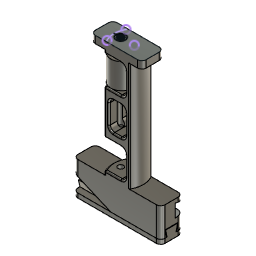
dual_mount_rolling_spool (Autodesk Fusion 360 design; units mm, degrees)
Autodesk Fusion 360 part; units mm, degrees
note: some values were not read from the file. Chosen so that the rebuilt part matches the saved one: which face or edge a step refers to.
sketch "Sketch1" plane through (0, 0, 0) normal (0, 0, 1) x (1, 0, 0)
  line L0 (0, 0) -> (60, 0)
  line L1 (60, 0) -> (60, 15)
  line L2 (60, 15) -> (0, 15)
  line L3 (0, 15) -> (0, 0)
  dimension "d1" = 60
  dimension "d2" = 15
  constraint horizontal L0
  constraint vertical L1
  constraint horizontal L2
  constraint vertical L3
  constraint coincident L0.start L3.end
  measures "d1" distance of L0.start L0.end
  measures "d2" distance of L0.start L2.end
extrude "Extrude1" add sketch "Sketch1" along normal blind 10 makes body 1
sketch "Sketch2" plane through (0, 0, 10) normal (0, 0, 1) x (-1, 0, 0)
  line L0 (0, -15) -> (0, 0)
  line L1 (0, 0) -> (-60, 0)
  line L2 (-60, 0) -> (-60, -15)
  line L3 (-60, -15) -> (0, -15)
  line L4 (-40.5, 0) -> (-19.5, 0)
  line L5 (-19.5, 0) -> (-19.5, -15)
  line L6 (-19.5, -15) -> (-40.5, -15)
  line L7 (-40.5, -15) -> (-40.5, 0) construction
  line L8 (-40.5, 0) -> (-19.5, -15) construction
  line L9 (-19.5, 0) -> (-40.5, -15) construction
  line L10 (-38.4665, -15) -> (-38.4665, 0) construction
  arc A0 (-38.4665, 0) -> (-38.4665, -15) centre (-25.6527, -7.5) ccw
  line L11 (-30, -7.5) -> (-30, -10.6) construction
  arc A1 (-21.5335, -15) -> (-21.5335, 0) centre (-34.3473, -7.5) ccw
  point P0 (-30, -7.5)
  dimension "d5" = 21
  constraint horizontal L4
  constraint perpendicular L4 L5
  constraint parallel L4 L6
  constraint parallel L5 L7
  constraint coincident L8 P0
  constraint coincident L9 P0
  constraint vertical L10
  constraint coincident L6 L10.start
  constraint coincident L3 L10.start
  constraint coincident L4 L10.end
  constraint coincident L1 L10.end
  constraint tangent L7 A0
  constraint coincident P0 L11.start
  constraint vertical L11
  constraint symmetric L10.start L11 A1.start
  constraint symmetric L10.end L11 A1.end
  constraint symmetric A0 L11 A1
  measures "d5" distance of L5.end L6.end
extrude "Extrude2" add sketch "Sketch2" along normal blind 75 contours L1 L3 L4 L6 A0 A1 bodies 1
fillet "Fillet1" radius 1 4 edges at (38.4665, 15, 47.5) (21.5335, 15, 47.5) (38.4665, 0, 47.5) (21.5335, 0, 47.5) on bodies 1
fillet "Fillet2" radius 3 4 edges at (60, 15, 5) (60, 0, 5) (0, 15, 5) (0, 0, 5) on bodies 1
sketch "Sketch3" plane through (0, 15, 0) normal (0, 1, 0) x (-1, 0, 0)
  line L0 (-3, 0) -> (-3, 10)
  line L1 (-3, 10) -> (-22.1204, 10)
  line L2 (-22.1204, 10) -> (-22.1204, 85)
  line L3 (-22.1204, 85) -> (-37.8796, 85)
  line L4 (-37.8796, 85) -> (-37.8796, 10)
  line L5 (-37.8796, 10) -> (-57, 10)
  line L6 (-57, 10) -> (-57, 0)
  line L7 (-57, 0) -> (-3, 0)
  line L8 (-22.1204, 10) -> (-22.1204, 35) construction
  line L9 (-22.1204, 35) -> (-22.1204, 60) construction
  line L10 (-27.4, 37.8) -> (-32.6, 37.8)
  line L11 (-35.6, 40.8) -> (-35.6, 54.2)
  line L12 (-32.6, 57.2) -> (-27.4, 57.2)
  line L13 (-24.4, 54.2) -> (-24.4, 40.8)
  line L14 (-24.4, 37.8) -> (-35.6, 57.2) construction
  line L15 (-35.6, 37.8) -> (-24.4, 57.2) construction
  arc A0 (-32.6, 57.2) -> (-35.6, 54.2) centre (-32.6, 54.2) ccw
  arc A1 (-24.4, 54.2) -> (-27.4, 57.2) centre (-27.4, 54.2) ccw
  arc A2 (-35.6, 40.8) -> (-32.6, 37.8) centre (-32.6, 40.8) ccw
  arc A3 (-27.4, 37.8) -> (-24.4, 40.8) centre (-27.4, 40.8) ccw
  line L16 (-22.1204, 35) -> (-24.6, 35) construction
  line L17 (-22.1204, 60) -> (-24.4, 60) construction
  line L18 (-24.4, 65.8) -> (-24.4, 79.2)
  arc A4 (-27.4, 62.8) -> (-24.4, 65.8) centre (-27.4, 65.8) ccw
  line L19 (-32.6, 62.8) -> (-27.4, 62.8)
  arc A5 (-35.6, 65.8) -> (-32.6, 62.8) centre (-32.6, 65.8) ccw
  line L20 (-35.6, 79.2) -> (-35.6, 65.8)
  arc A6 (-32.6, 82.2) -> (-35.6, 79.2) centre (-32.6, 79.2) ccw
  line L21 (-27.4, 82.2) -> (-32.6, 82.2)
  arc A7 (-24.4, 79.2) -> (-27.4, 82.2) centre (-27.4, 79.2) ccw
  line L22 (-27.4, 32.2) -> (-32.6, 32.2)
  arc A8 (-24.4, 29.2) -> (-27.4, 32.2) centre (-27.4, 29.2) ccw
  line L23 (-24.4, 15.8) -> (-24.4, 29.2)
  arc A9 (-32.6, 32.2) -> (-35.6, 29.2) centre (-32.6, 29.2) ccw
  line L24 (-35.6, 29.2) -> (-35.6, 15.8)
  line L25 (-32.6, 12.8) -> (-27.4, 12.8)
  arc A10 (-27.4, 12.8) -> (-24.4, 15.8) centre (-27.4, 15.8) ccw
  arc A11 (-35.6, 15.8) -> (-32.6, 12.8) centre (-32.6, 15.8) ccw
  line L26 (-19.5, 85) -> (-21.2374, 85)
  line L27 (-19.5, 85) -> (-19.5, 10)
  line L28 (-30, 12.8) -> (-19.5, 12.8)
  line L29 (-30, 32.2) -> (-19.5, 32.2)
  line L30 (-19.5, 12.8) -> (-19.5, 32.2)
  line L31 (-30, 62.8) -> (-19.5, 62.8)
  line L32 (-30, 82.2) -> (-19.5, 82.2)
  point P0 (-30, 47.5)
  dimension "d12" = 25
  dimension "d13" = 25
  dimension "d14" = 3
  dimension "d15" = 3
  dimension "d16" = 3
  dimension "d17" = 3
  constraint coincident L1.end L2.start
  constraint perpendicular L3 L8
  constraint parallel L2 L9
  constraint horizontal L10
  constraint perpendicular L10 L11
  constraint parallel L10 L12
  constraint parallel L11 L13
  constraint coincident L14 P0
  constraint coincident L15 P0
  constraint coincident L14.end L12
  constraint coincident L14.end L11
  constraint tangent L12 A0
  constraint tangent L11 A0
  constraint coincident L15.end L12
  constraint coincident L15.end L13
  constraint tangent L12 A1
  constraint tangent L13 A1
  constraint coincident L15.start L11
  constraint coincident L15.start L10
  constraint tangent L11 A2
  constraint tangent L10 A2
  constraint coincident L14.start L13
  constraint coincident L14.start L10
  constraint tangent L13 A3
  constraint tangent L10 A3
  constraint perpendicular L2 L16
  constraint perpendicular L2 L17
  constraint symmetric L12.start L17 L19.start
  constraint symmetric L11.end L17 A5.start
  constraint symmetric A0 L17 A5
  constraint symmetric L12.end L17 A4.start
  constraint symmetric L13.start L17 L18.start
  constraint symmetric A1 L17 A4
  constraint symmetric L11.start L17 L20.start
  constraint symmetric L10.end L17 A6.start
  constraint symmetric A2 L17 A6
  constraint symmetric L13.end L17 L18.end
  constraint symmetric L10.start L17 L21.start
  constraint symmetric A3 L17 A7
  constraint symmetric L12.start L16 L25.start
  constraint symmetric L11.end L16 L24.end
  constraint symmetric A0 L16 A11
  constraint symmetric L12.end L16 L25.end
  constraint symmetric L13.start L16 L23.start
  constraint symmetric A1 L16 A10
  constraint symmetric L11.start L16 A9.end
  constraint symmetric L10.end L16 L22.end
  constraint symmetric A2 L16 A9
  constraint symmetric L13.end L16 A8.start
  constraint symmetric L10.start L16 L22.start
  constraint symmetric A3 L16 A8
  constraint coincident L26.start L27.start
  constraint coincident L1 L27.end
  constraint perpendicular L1 L27
  constraint midpoint L25 L28.start
  constraint coincident L27 L28.end
  constraint perpendicular L27 L28
  constraint midpoint L22 L29.start
  constraint coincident L27 L29.end
  constraint perpendicular L27 L29
  constraint midpoint L19 L31.start
  constraint coincident L27 L31.end
  constraint perpendicular L27 L31
  constraint midpoint L21 L32.start
  constraint coincident L27 L32.end
  constraint perpendicular L27 L32
  measures "d12" distance of L1.end L8.end
  measures "d13" distance of L8.end L9.end
  measures "d14" radius of A0
  measures "d15" radius of A1
  measures "d16" radius of A2
  measures "d17" radius of A3
extrude "Extrude6" cut sketch "Sketch3" against normal blind 15 contours L2 L27 L28 L29 L30 | L2 A8 L23 A10 L28 L29 | L2 L27 L31 L32 | L2 L18 A4 A7 L31 L32 bodies 1
extrude "Extrude3" cut sketch "Sketch3" against normal blind 15 contours L22 A8 L23 A9 L24 L25 A10 A11 L28 L29 | L18 A4 L19 A5 L20 A6 L21 A7 L31 L32 | L10 L11 L12 L13 A0 A1 A2 A3 bodies 1
fillet "Fillet3" radius 1 48 edges at (27.3602, 15, 82.2) (34.7213, 15, 81.3213) (35.6, 15, 72.5) (34.7213, 15, 63.6787) (27.3602, 15, 62.8) (27.3602, 15, 32.2) (34.7213, 15, 31.3213) (35.6, 15, 22.5) (34.7213, 15, 13.6787) (27.3602, 15, 12.8) (30, 15, 37.8) (25.2787, 15, 38.6787) (24.4, 15, 47.5) (25.2787, 15, 56.3213) (30, 15, 57.2) (34.7213, 15, 56.3213) (35.6, 15, 47.5) (34.7213, 15, 38.6787) (21.6053, 14.8571, 12.8) (21.6053, 0.1429, 12.8) (19.5, 7.5, 12.8) (27.3602, 0, 12.8) (34.7213, 0, 13.6787) (35.6, 0, 22.5) (34.7213, 0, 31.3213) (21.6053, 14.8571, 32.2) (19.5, 7.5, 32.2) (21.6053, 0.1429, 32.2) (27.3602, 0, 32.2) (21.6053, 14.8571, 62.8) (27.3602, 0, 62.8) (21.6053, 0.1429, 62.8) (19.5, 7.5, 62.8) (34.7213, 0, 63.6787) (35.6, 0, 72.5) (34.7213, 0, 81.3213) (21.6053, 14.8571, 82.2) (19.5, 7.5, 82.2) (21.6053, 0.1429, 82.2) (27.3602, 0, 82.2) (30, 0, 37.8) (34.7213, 0, 38.6787) (35.6, 0, 47.5) (34.7213, 0, 56.3213) (30, 0, 57.2) (25.2787, 0, 56.3213) (24.4, 0, 47.5) (25.2787, 0, 38.6787) on bodies 1
sketch "Sketch4" plane through (0, 0, 10) normal (0, 0, 1) x (-1, 0, 0)
  arc A0 (-57, 0) -> (-60, -3) centre (-57, -3) ccw
  line L0 (-60, -3) -> (-60, -12)
  arc A1 (-60, -12) -> (-57, -15) centre (-57, -12) ccw
  line L1 (-57, -15) -> (-37.8796, -15)
  arc A2 (-38.7626, -14.4694) -> (-37.8796, -15) centre (-37.8796, -14) ccw
  arc A3 (-38.7626, -0.5306) -> (-38.7626, -14.4694) centre (-25.6527, -7.5) ccw
  arc A4 (-37.8796, 0) -> (-38.7626, -0.5306) centre (-37.8796, -1) ccw
  line L2 (-37.8796, 0) -> (-57, 0)
  line L3 (-60, -7.5) -> (-55, -7.5)
  circle A5 centre (-51.8, -7.5) radius 3.2
  circle A6 centre (-51.8, -7.5) radius 1.9
  dimension "d22" = 5
  dimension "d23" = 6.4
  dimension "d24" = 3.8
  constraint midpoint L0 L3.start
  constraint perpendicular L0 L3
  constraint coincident L3.end A5
  constraint concentric A5 A6
  measures "d22" distance of L3.start L3.end
  measures "d23" diameter of A5
  measures "d24" diameter of A6
extrude "Extrude4" [suppressed]
extrude "Extrude5" [suppressed]
ref_plane "WorkPlane1" through (30, 7.5, 5) normal (1, 0, 0) x (0, 1, 0)
mirror "Mirror1" [suppressed]
sketch "Sketch5" plane through (0, 0, 85) normal (0, 0, 1) x (-1, 0, 0)
  arc A0 (-21.2374, -0.5306) -> (-22.1204, 0) centre (-22.1204, -1) ccw
  line L0 (-22.1204, 0) -> (-37.8796, 0)
  arc A1 (-37.8796, 0) -> (-38.7626, -0.5306) centre (-37.8796, -1) ccw
  arc A2 (-38.7626, -0.5306) -> (-38.7626, -14.4694) centre (-25.6527, -7.5) ccw
  arc A3 (-38.7626, -14.4694) -> (-37.8796, -15) centre (-37.8796, -14) ccw
  line L1 (-37.8796, -15) -> (-22.1204, -15)
  arc A4 (-22.1204, -15) -> (-21.2374, -14.4694) centre (-22.1204, -14) ccw
  arc A5 (-21.2374, -14.4694) -> (-21.2374, -0.5306) centre (-34.3473, -7.5) ccw
  line L2 (-30, -15) -> (-47, -15)
  line L3 (-44, -15) -> (-15, -15)
  line L4 (-12, -12) -> (-12, -3)
  line L5 (-15, 0) -> (-44, 0)
  line L6 (-47, -3) -> (-47, -12)
  arc A6 (-15, -15) -> (-12, -12) centre (-15, -12) ccw
  arc A7 (-12, -3) -> (-15, 0) centre (-15, -3) ccw
  arc A8 (-47, -12) -> (-44, -15) centre (-44, -12) ccw
  arc A9 (-44, 0) -> (-47, -3) centre (-44, -3) ccw
  point P0 (-12, -15)
  dimension "d34" = 17
  dimension "d35" = 35
  dimension "d36" = 3
  dimension "d37" = 3
  dimension "d38" = 3
  dimension "d39" = 3
  constraint midpoint L1 L2.start
  constraint parallel L1 L2
  constraint horizontal L3
  constraint vertical L4
  constraint horizontal L5
  constraint vertical L6
  constraint coincident P0 L3
  constraint coincident P0 L4
  constraint tangent L3 A6
  constraint tangent L4 A6
  constraint tangent L4 A7
  constraint tangent L5 A7
  constraint coincident L2.end L6
  constraint coincident L2.end L3
  constraint tangent L6 A8
  constraint tangent L3 A8
  constraint tangent L6 A9
  constraint tangent L5 A9
  measures "d34" distance of L2.start L2.end
  measures "d35" distance of L2.end P0
  measures "d36" radius of A6
  measures "d37" radius of A7
  measures "d38" radius of A8
  measures "d39" radius of A9
extrude "Extrude7" add sketch "Sketch5" along normal blind 5 bodies 1
sketch "Sketch6" plane through (0, 0, 90) normal (0, 0, 1) x (-1, 0, 0)
  arc A0 (-44, 0) -> (-47, -3) centre (-44, -3) ccw
  line L0 (-47, -3) -> (-47, -12)
  arc A1 (-47, -12) -> (-44, -15) centre (-44, -12) ccw
  line L1 (-44, -15) -> (-15, -15)
  arc A2 (-15, -15) -> (-12, -12) centre (-15, -12) ccw
  line L2 (-12, -12) -> (-12, -3)
  arc A3 (-12, -3) -> (-15, 0) centre (-15, -3) ccw
  line L3 (-15, 0) -> (-44, 0)
  arc A4 (-22.1204, -14) -> (-22.1204, -1) centre (-34.3473, -7.5) ccw
  line L4 (-20.5, -7.5) -> (-25, -7.5)
  circle A5 centre (-25, -7.5) radius 1.9
  circle A6 centre (-25, -7.5) radius 3.2
  dimension "d42" = 4.5
  dimension "d43" = 3.8
  dimension "d44" = 6.4
  constraint midpoint A4 L4.start
  constraint horizontal L4
  constraint coincident L4.end A5.centre
  measures "d42" distance of L4.start L4.end
  measures "d43" diameter of A5
  measures "d44" diameter of A6
extrude "Extrude8" cut sketch "Sketch6" against normal blind 90 contours A5 bodies 1
extrude "Extrude9" cut sketch "Sketch6" against normal blind 1.5 contours A6 bodies 1
sketch "Sketch7" plane through (0, 0, 0) normal (0, 0, -1) x (1, 0, 0)
  circle A0 centre (25, -7.5) radius 1.9
  arc A1 (3, 0) -> (0, -3) centre (3, -3) ccw
  line L0 (0, -3) -> (0, -12)
  arc A2 (0, -12) -> (3, -15) centre (3, -12) ccw
  line L1 (3, -15) -> (57, -15)
  arc A3 (57, -15) -> (60, -12) centre (57, -12) ccw
  line L2 (60, -12) -> (60, -3)
  arc A4 (60, -3) -> (57, 0) centre (57, -3) ccw
  line L3 (57, 0) -> (3, 0)
  circle A5 centre (25, -7.5) radius 3.2
  dimension "d49" = 6.4
  constraint concentric A0 A5
  measures "d49" diameter of A5
extrude "Extrude10" [suppressed]
sketch "Sketch8" plane through (0, 0, 0) normal (1, 0, 0) x (0, 1, 0)
  line L0 (1, 62.8) -> (14, 62.8)
  line L1 (14, 57.2) -> (1, 57.2)
  line L2 (7.5, 57.2) -> (7.5, 62.8) construction
  line L3 (4.65, 61.6) -> (10.35, 61.6)
  line L4 (10.35, 61.6) -> (10.35, 58.4)
  line L5 (10.35, 58.4) -> (4.65, 58.4)
  line L6 (4.65, 58.4) -> (4.65, 61.6)
  line L7 (4.65, 61.6) -> (10.35, 58.4) construction
  line L8 (10.35, 61.6) -> (4.65, 58.4) construction
  point P0 (7.5, 60)
  dimension "d52" = 5.7
  dimension "d53" = 3.2
  constraint midpoint L1 L2.start
  constraint midpoint L0 L2.end
  constraint horizontal L3
  constraint perpendicular L3 L4
  constraint parallel L3 L5
  constraint parallel L4 L6
  constraint coincident L7 P0
  constraint coincident L8 P0
  constraint midpoint L2 P0
  measures "d52" distance of L4.end L5.end
  measures "d53" distance of L3.end L4.end
extrude "Extrude11" cut sketch "Sketch8" along normal blind 28.9 bodies 1
ref_plane "WorkPlane2" through (25.6324, 7.5, 47.5) normal (0, 0, 1) x (-1, 0, 0)
mirror "Mirror2" about plane through (25.6324, 7.5, 47.5) normal (0, 0, 1) of "Extrude11"
ref_plane "WorkPlane3" through (25.6324, 7.5, 63.8) normal (0, 0, 1) x (-1, 0, 0)
sketch "Sketch9" plane through (25.6324, 7.5, 63.8) normal (0, 0, 1) x (1, 0, 0)
  circle A0 centre (0, 0) radius 7.5
  circle A1 centre (0, 0) radius 2
  dimension "d60" = 15
  dimension "d61" = 4
  constraint coincident A0.centre A1.centre
  constraint concentric A0 A1
  measures "d60" diameter of A0
  measures "d61" diameter of A1
extrude "Extrude12" add sketch "Sketch9" along normal blind 17.4 separate body makes body 2
extrude "Extrude13" add 1 faces at (46.9667, 7.5, 0) along direction (0, 0, -1) blind 10 on bodies 1 bodies 1
sketch "Sketch10" plane through (0, 0, 0) normal (-1, 0, 0) x (0, -1, 0)
  line L0 (-3, -10) -> (-3, 10)
  line L1 (-3, 10) -> (-12, 10)
  line L2 (-12, 10) -> (-12, -10)
  line L3 (-12, -10) -> (-3, -10)
  line L4 (-12, -10) -> (-12, -5) construction
  line L5 (-12, -5) -> (-3, -5)
  line L6 (-3, -5) -> (-4.1123, -10)
  line L7 (-3.3, -5) -> (-4.4123, -10)
  line L8 (-12, -5.3) -> (-3, -5.3)
  line L9 (-7.5, -5) -> (-7.5, -0.8) construction
  line L10 (-11.7, -5) -> (-10.5877, -10)
  line L11 (-12, -5) -> (-10.8877, -10)
  line L12 (-10.0561, -1.5561) -> (-15.0561, -0.4439)
  line L13 (-10.0561, 7.4439) -> (-10.0561, -1.5561)
  line L14 (-10.0561, 7.4439) -> (-15.0561, 6.3316)
  line L15 (-15.0561, -0.4439) -> (-15.0561, 6.3316)
  dimension "d66" = 5
  constraint coincident L2.end L3.start
  constraint perpendicular L3 L4
  constraint coincident L0 L5.end
  constraint perpendicular L0 L5
  constraint coincident L3 L6.end
  constraint midpoint L5 L9.start
  constraint perpendicular L8 L9
  constraint symmetric L5.end L9 L4.end
  constraint symmetric L6.end L9 L11.end
  constraint symmetric L7.start L9 L10.start
  constraint symmetric L7.end L9 L10.end
  constraint vertical L15
  measures "d66" distance of L2.end L4.end
extrude "Extrude16" add 1 faces at (46.9667, 7.5, -10) along direction (0, 0, -1) blind 3 separate body on bodies 1 makes body 3
extrude "Extrude14" cut sketch "Sketch10" against normal blind 60 contours L3 L6 L7 L8 | L5 L6 L7 L8 | L3 L7 L8 L10 | L5 L7 L8 L10 | L3 L8 L10 L11 | L5 L8 L10 L11 | L2 L12 L13 L14 | L2 L12 L14 L15 bodies 1
sketch "Sketch11" plane through (0, 0, -5) normal (0, 0, -1) x (1, 0, 0)
  circle A0 centre (25, -7.5) radius 1.9
  line L0 (0, -3) -> (0, -12)
  line L1 (0, -12) -> (60, -12)
  line L2 (60, -12) -> (60, -3)
  line L3 (60, -3) -> (0, -3)
  circle A1 centre (25, -7.5) radius 3.2
  dimension "d69" = 6.4
  constraint concentric A0 A1
  measures "d69" diameter of A1
extrude "Extrude15" cut sketch "Sketch11" against normal blind 15 contours A1 bodies 1
extrude "Extrude17" add sketch "Sketch10" against normal blind 60 contours L3 L7 L8 L10 bodies 3
sketch "Sketch12" plane through (0, 0, -5.3) normal (0, 0, 1) x (-1, 0, 0)
  line L0 (0, -11.6333) -> (0, -3.3667)
  line L1 (0, -3.3667) -> (-60, -3.3667)
  line L2 (-60, -3.3667) -> (-60, -11.6333)
  line L3 (-60, -11.6333) -> (0, -11.6333)
  line L4 (0, -7.5) -> (-8, -7.5)
  circle A0 centre (-8, -7.5) radius 3.2
  circle A1 centre (-8, -7.5) radius 1.9
  dimension "d76" = 8
  dimension "d77" = 6.4
  dimension "d78" = 3.8
  constraint midpoint L0 L4.start
  constraint perpendicular L0 L4
  constraint coincident L4.end A0.centre
  constraint concentric A0 A1
  measures "d76" distance of L4.start L4.end
  measures "d77" diameter of A0
  measures "d78" diameter of A1
extrude "Extrude18" cut sketch "Sketch12" against normal blind 7.7 contours A1 bodies 3
extrude "Extrude19" cut sketch "Sketch12" against normal blind 2 contours A0 bodies 3
mirror "Mirror3" about plane through (30, 7.5, 5) normal (1, 0, 0) of "Extrude18", "Extrude19"
extrude "Extrude20" cut sketch "Sketch6" against normal blind 103 contours A5 bodies 2 3
sketch "Sketch13" plane through (0, 15, 0) normal (0, 1, 0) x (-1, 0, 0)
  line L0 (-3, -0.4563) -> (-57, -0.4563)
  line L1 (-57, -0.4563) -> (-57, -10)
  line L2 (-57, -10) -> (-3, -10)
  line L3 (-3, -10) -> (-3, -0.4563)
  line L4 (0, 7.4439) -> (0, -1.5561)
  line L5 (0, 1) -> (-25.5865, -10)
  line L6 (0, 1) -> (0, -10)
  line L7 (0, -10) -> (-25.5865, -10)
  constraint coincident L4 L5.start
  constraint coincident L2 L5.end
  constraint perpendicular L2 L6
  constraint perpendicular L4 L7
extrude "Extrude21" cut sketch "Sketch13" against normal blind 15 contours L0 L2 L3 L5 L7 | L0 L3 L4 L5 L6 L7 bodies 1
fillet "Fillet4" radius 0.5 1 edges at (4.6666, 12.5281, -1.0062) on bodies 1
equation "d12 = 75.000 mm / 3"
equation "d42 = 7.5 mm - 3 mm"
equation "d54 = 26.90 mm + 2 mm"
equation "d56 = -30.60 mm / 2"
equation "d62 = 18.40 mm - 1 mm"
